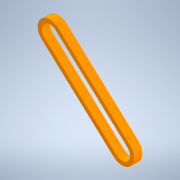
# Autodesk Inventor part: 슬롯
Saved by Autodesk Inventor 2022 (Build 260153000, 153)
## iProperties
Created: 2022-10-28
Part Number: 슬롯
Material: 일반
Document SubType Name: Modeling
Designer: whdls
Density: 1 g/cm^3
Appearance: 기본값
Author: whdls
Autodesk Inventor part; units mm, degrees
ref_plane "YZ Plane" through (0, 0, 0) normal (1, 0, 0) x (0, 1, 0)
ref_plane "XZ Plane" through (0, 0, 0) normal (0, 1, 0) x (-1, 0, 0)
ref_plane "XY Plane" through (0, 0, 0) normal (0, 0, 1) x (1, 0, 0)
sketch "스케치2" plane through (0, 0, 0) normal (0, 0, 1) x (1, 0, 0)
  circle A0 centre (0, 0) radius 1 projected
  circle A1 centre (-8.8212, 8.0626) radius 1 projected
  line L0 (-0.6747, -0.7381) -> (-9.4959, 7.3245)
  line L1 (0.6747, 0.7381) -> (-8.1466, 8.8007)
  line L2 (-1.012, -1.1072) -> (-9.8332, 6.9554)
  line L3 (1.012, 1.1072) -> (-7.8092, 9.1698)
  circle A2 centre (0, 0) radius 1.5
  circle A3 centre (-8.8212, 8.0626) radius 1.5
  dimension "d0" = 0.5
  dimension "d1" = 0.5
  dimension "d2" = 0.5
  dimension "d3" = 0.5
  constraints: 8 end point, 4 point on circle, 4 tangent, 2 centre point, 2 parallel
  measures "d0" distance between parallel lines of L0 L2
  measures "d1" distance between parallel lines of L1 L3
  measures "d2" radial gap between concentric circles of A3 A1
  measures "d3" radial gap between concentric circles of A2 A0
extrude "돌출1" add sketch "스케치2" against normal blind 1 contours A0 L1 A2 L0 | L1 A3 L3 A2 | A2 L2 A3 L0 | L1 A1 L0 A3 picked at (0.2294, 1.2405) picked at (-9.0506, 6.8221)
